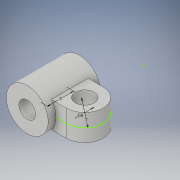
# Autodesk Inventor part: 避震器上部
Saved by Autodesk Inventor 2019 (Build 230136000, 136)
## iProperties
Created: 2020-03-20
Part Number: 避震器上部
Material: 一般
Document SubType Name: Modeling
Designer: 黃柏維
Density: 1 g/cm^3
Appearance: 預設
Author: 黃柏維
Autodesk Inventor part; units mm, degrees
ref_plane "YZ Plane" through (0, 0, 0) normal (1, 0, 0) x (0, 1, 0)
ref_plane "XZ Plane" through (0, 0, 0) normal (0, 1, 0) x (-1, 0, 0)
ref_plane "XY Plane" through (0, 0, 0) normal (0, 0, 1) x (1, 0, 0)
sketch "草圖2" plane through (0, 0, 0) normal (0, 0, 1) x (1, 0, 0)
  circle A0 centre (0, 0) radius 1.6
  circle A1 centre (0, 0) radius 4
  dimension "d6" = 3.2
  dimension "d7" = 8
  constraints: 2 centre point, 2 coincident
  measures "d6" diameter of A0
  measures "d7" diameter of A1
extrude "擠出2" add sketch "草圖2" along normal blind 10
sketch "草圖3" plane through (0, 0, 0) normal (0, 1, 0) x (-1, 0, 0)
  line L0 (0, 2.5) -> (0, 7.5)
  circle A0 centre (-6, 5) radius 1.8
  line L1 (-3, 2.5) -> (-3, 7.5)
  circle A1 centre (-6, 5) radius 3.5
  line L2 (-6, 1.5) -> (0, 1.5)
  line L3 (-6, 8.5) -> (0, 8.5)
  line L4 (0, 8.5) -> (0, 1.5)
  point P0 (0, 0)
  point P1 (-3.8558, -8.4985)
  dimension "d10" = 5
  dimension "d13" = 3.6
  dimension "d16" = 7
  constraints: 10 end point, 2 centre point, 2 horizontal, 2 point on circle, 1 coincident, 1 perpendicular, 1 vertical
  measures "d10" distance of L0.start L0.end
  measures "d13" diameter of A0
  measures "d16" diameter of A1
extrude "Extrusion4" add sketch "草圖3" along normal mid plane 5
sketch "Sketch5" plane through (0, 0, 8.5) normal (0, 0, 1) x (1, 0, 0)
  circle A0 centre (0, 0) radius 1.6
  dimension "d19" = 3.2
  constraints: 1 centre point, 1 coincident
  measures "d19" diameter of A0
extrude "Extrusion5" cut sketch "Sketch5" along normal through all both and the other way through all
